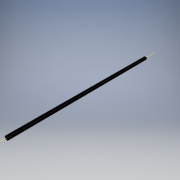
# Autodesk Inventor part: Profile-Square#16
Saved by Autodesk Inventor 2018 (Build 220112000, 112)
## iProperties
Created: 2025-02-17
Part Number: Profile-Square#16
Material: Všeobecné
Document SubType Name: Modeling
Designer: Jozko Mrkvicka
Density: 1 g/cm^3
Appearance: Výchozí
Author: Jozko Mrkvicka
Autodesk Inventor part; units mm, degrees
ref_plane "YZ Plane" through (0, 0, 0) normal (1, 0, 0) x (0, 1, 0)
ref_plane "XZ Plane" through (0, 0, 0) normal (0, 1, 0) x (-1, 0, 0)
ref_plane "XY Plane" through (0, 0, 0) normal (0, 0, 1) x (1, 0, 0)
sketch "Náčrt1" plane through (0, 0, 0) normal (0, 0, 1) x (1, 0, 0)
  line L0 (-15, -15) -> (15, -15)
  line L1 (15, -15) -> (15, 15)
  line L2 (15, 15) -> (-15, 15)
  line L3 (-15, 15) -> (-15, -15)
  line L4 (-15, -15) -> (15, 15) construction
  line L5 (15, -15) -> (-15, 15) construction
  line L6 (-13, -13) -> (13, -13)
  line L7 (13, -13) -> (13, 13)
  line L8 (13, 13) -> (-13, 13)
  line L9 (-13, 13) -> (-13, -13)
  line L10 (-13, -13) -> (13, 13) construction
  line L11 (13, -13) -> (-13, 13) construction
  point P0 (0, 0)
  dimension "d0" = 30
  dimension "d1" = 30
  dimension "d2" = 26
  dimension "d3" = 26
  constraints: 24 end point, 4 midpoint, 4 parallel, 2 horizontal, 2 perpendicular
  measures "d0" distance of L2.end L1.end
  measures "d1" distance of L1.end L0.end
  measures "d2" distance of L8.end L7.end
  measures "d3" distance of L8.end L6.start
extrude "Vysunutí1" add sketch "Náčrt1" along normal blind 1790
sketch "Náčrt2" plane through (-15, 15, 0) normal (0, 1, 0) x (1, 0, 0)
  circle A0 centre (15, -15) radius 1.5
  line L0 (30, 0) -> (0, 0) projected
  line L1 (0, 0) -> (0, -1790) projected
  line L2 (30, -1790) -> (0, -1790) projected
  line L3 (30, 0) -> (30, -1790) projected
  point P0 (15, 0)
  dimension "d8" = 3
  dimension "d13" = 15
  dimension "d19" = 15
  constraints: 1 centre point
  measures "d8" diameter of A0
  measures "d13" distance from line of L0 A0.centre
  measures "d19" distance from line of L1 A0.centre
extrude "Vysunutí2" cut sketch "Náčrt2" against normal up to surface (2 mm away) contours A0
sketch "Náčrt3" plane through (-15, -15, 0) normal (0, -1, 0) x (1, 0, 0)
  line L0 (30, 0) -> (0, 0) projected
  line L1 (0, 0) -> (0, 1790) projected
  line L2 (30, 1790) -> (0, 1790) projected
  line L3 (30, 0) -> (30, 1790) projected
  circle A0 centre (15, 15) radius 1.5 projected
  circle A1 centre (15, 15) radius 5
  point P0 (15, 0)
  dimension "d15" = 10
  constraints: 1 centre point, 1 coincident
  measures "d15" diameter of A1
extrude "Vysunutí3" cut sketch "Náčrt3" against normal up to surface (2 mm away) contours A0 | A1
pattern_linear "Obdélníkové pole1" count 6 spacing 293 along (0, 0, 1) of "Vysunutí2"
pattern_linear "Obdélníkové pole3" count 6 spacing 293 along (0, 0, 1) of "Vysunutí3"
equation "\"d0\" = width"
equation "\"d1\" = width"
equation "\"d2\" = width - 2 * thickness"
equation "\"d3\" = width - 2 * thickness"
equation "\"d4\" = length"
equation "\"d8\" = holeDia"
equation "\"d13\" = holeOffset"
equation "\"d19\" = 0.5 * width"
equation "\"d15\" = holeDiaOpposite"
equation "\"d22\" = holeDistance"
equation "\"d28\" = holeDistance"
equation "\"width\" = gSquareProfile_Width_Rack"
equation "\"thickness\" = gSquareProfile_Thickness_Rack"
equation "\"length\" = gRack_Rom_Height - 2 * width"
equation "\"holeDistance\" = 293"
equation "\"holeDiaOpposite\" = 10"
equation "\"holeDia\" = 3"
equation "\"holeOffset\" = 0.5 * width"
equation "\"gSquareProfile_Width_Rack\" = 30"
equation "\"gSquareProfile_Thickness_Rack\" = 2"
equation "\"gRack_Rom_Height\" = 1850"
